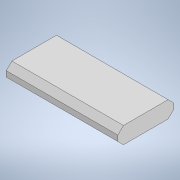
# Autodesk Inventor part: lipol-40mAh
Saved by Autodesk Inventor 2022.3 (Build 263350000, 350)
## iProperties
Created: 2022-12-14
Part Number: lipol-40mAh
Material: Generic
Document SubType Name: Modeling
Designer: komputer
Density: 1 g/cm^3
Appearance: Default
Author: komputer
Autodesk Inventor part; units mm, degrees
ref_plane "YZ Plane" through (0, 0, 0) normal (1, 0, 0) x (0, 1, 0)
ref_plane "XZ Plane" through (0, 0, 0) normal (0, 1, 0) x (-1, 0, 0)
ref_plane "XY Plane" through (0, 0, 0) normal (0, 0, 1) x (1, 0, 0)
sketch "Sketch1" plane through (0, 0, 0) normal (0, 1, 0) x (-1, 0, 0)
  line L0 (7.294, 10.1667) -> (-12.706, 10.1667)
  line L1 (-12.706, 10.1667) -> (-12.706, 0.1667)
  line L2 (-12.706, 0.1667) -> (7.294, 0.1667)
  line L3 (7.294, 0.1667) -> (7.294, 10.1667)
  point P0 (0, 0)
  dimension "d0" = 20
  dimension "d1" = 10
  constraints: 8 end point, 2 parallel, 1 horizontal, 1 perpendicular
  measures "d0" distance of L2.end L1.end
  measures "d1" distance of L1.end L0.end
extrude "Extrusion1" add sketch "Sketch1" along normal blind 3
chamfer "Chamfer1" distance 1 angle 45 4 edges at (2.706, 3, 10.1667) (2.706, 0, 10.1667) (2.706, 0, 0.1667) (2.706, 3, 0.1667)
body "Solid1"
